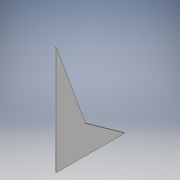
# Autodesk Inventor part: Rocket_MK_II_Fins_III
Saved by Autodesk Inventor 2017 (Build 210142000, 142)
## iProperties
Created: 2017-05-03
Part Number: Rocket_MK_II_Fins_III
Material: Generic
Document SubType Name: Modeling
Designer: Harrison
Density: 1 g/cm^3
Appearance: Default
Author: Harrison
Autodesk Inventor part; units mm, degrees
ref_plane "YZ Plane" through (0, 0, 0) normal (1, 0, 0) x (0, 1, 0)
ref_plane "XZ Plane" through (0, 0, 0) normal (0, 1, 0) x (-1, 0, 0)
ref_plane "XY Plane" through (0, 0, 0) normal (0, 0, 1) x (1, 0, 0)
sketch "Sketch1" plane through (0, 0, 0) normal (1, 0, 0) x (0, 1, 0)
  line L0 (0, 0) -> (120.65, 0)
  line L1 (0, 0) -> (0, -76.2)
  line L2 (120.65, 0) -> (31.4803, -32.2624)
  line L3 (31.4803, -32.2624) -> (0, -76.2)
  dimension "d0" = 120.65
  dimension "d1" = 76.2
  constraints: 8 end point, 1 horizontal, 1 vertical
  measures "d0" distance of L0.start L0.end
  measures "d1" distance of L0.start L1.end
extrude "Extrusion1" add sketch "Sketch1" along normal blind 1.27
body "Solid1"
